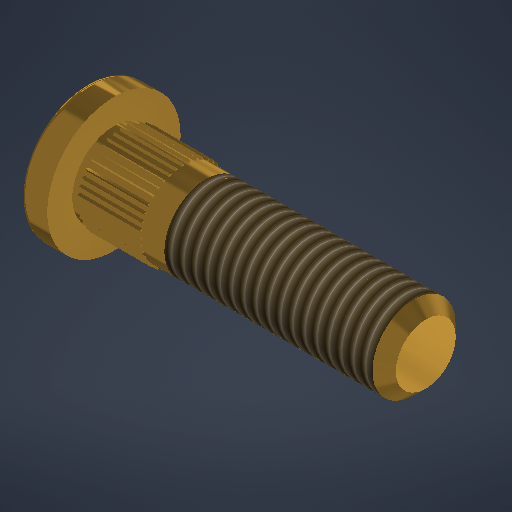
# Autodesk Inventor part: Lug Stud M12 X 45
Saved by Autodesk Inventor 2026.1 (Build 301233000, 233)
## iProperties
Created: 2015-03-25
Part Number: Lug Stud M12 X 45
Material: Generic
Document SubType Name: Modeling
Designer: Mohamed
Density: 1 g/cm^3
Appearance: Default
Author: Mohamed
Autodesk Inventor part; units mm, degrees
ref_plane "YZ Plane" through (0, 0, 0) normal (1, 0, 0) x (0, 1, 0)
ref_plane "XZ Plane" through (0, 0, 0) normal (0, 1, 0) x (-1, 0, 0)
sketch "Sketch1" plane through (0, 0, 0) normal (0, 0, 1) x (1, 0, 0)
  line L0 (0, 8.628) -> (0, 0)
  line L1 (0, 0) -> (49, 0)
  line L2 (49, 0) -> (49, 4.3276)
  line L3 (47.2899, 6) -> (4, 6)
  line L4 (4, 6) -> (4, 9.628)
  line L5 (1, 9.628) -> (4, 9.628)
  arc A0 (1, 9.628) -> (0, 8.628) centre (1, 8.628) ccw
  line L6 (47.2899, 6) -> (49, 4.3276)
  dimension "d0" = 6
  dimension "d3" = 1
  dimension "d4" = 4
  dimension "d17" = 45
  dimension "d18" = 1.7101
  dimension "d19" = 1.6724
  constraints: 14 end point, 4 perpendicular, 2 point on circle, 2 tangent, 1 centre point, 1 coincident, 1 parallel, 1 vertical
  measures "d0" distance between parallel lines of L1 L3
  measures "d3" radius of A0
  measures "d4" distance between parallel lines of L0 L4
  measures "d17" distance between parallel lines of L2 L4
  measures "d18" distance from line of L3.start L2
  measures "d19" vertical distance of L3.start L2.end
revolve "Revolution1" add sketch "Sketch1" angle 360 about axis through (0, 0, 0) along (1, 0, 0)
ref_plane "Work Plane1" through (14, 0, 0) normal (1, 0, 0) x (0, 0, -1)
sketch "Sketch2" plane through (14, 0, 0) normal (1, 0, 0) x (0, 0, -1)
  line L0 (0, 6.3282) -> (-0.2051, 5.9796)
  line L1 (0, 0) -> (0, 4.031)
  line L2 (0, 6.3282) -> (0.2051, 5.9796)
  arc A0 (0.2051, 5.9796) -> (-0.2051, 5.9796) centre (0, 0) ccw
  point P0 (0, 0)
  point P1 (-0.2227, 5.9496)
  point P2 (0.2227, 5.9496)
  constraints: 6 end point, 2 coincident, 2 point on circle, 1 centre point, 1 symmetric about line, 1 vertical
extrude "Extrusion1" add sketch "Sketch2" against normal blind 9
pattern_circular "Circular Pattern1" count 40 over 360 about axis through (1, 0, 0) along (1, 0, 0) of "Extrusion1"
thread "Thread2" size "M12x1.75" class "6g" standard "ANSI Metric M Profile" length 30
body "Solid1"
